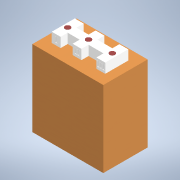
# Autodesk Inventor part: Mesa piezas
Saved by Autodesk Inventor 2020 (Build 240168000, 168)
## iProperties
Created: 2019-10-05
Part Number: Mesa piezas
Material: Genérico
Document SubType Name: Modeling
Designer: dasa1
Density: 1 g/cm^3
Appearance: Valor por defecto
Author: dasa1
Autodesk Inventor part; units mm, degrees
ref_plane "YZ Plane" through (0, 0, 0) normal (1, 0, 0) x (0, 1, 0)
ref_plane "XZ Plane" through (0, 0, 0) normal (0, 1, 0) x (-1, 0, 0)
ref_plane "XY Plane" through (0, 0, 0) normal (0, 0, 1) x (1, 0, 0)
sketch "Boceto1" plane through (0, 0, 0) normal (0, 1, 0) x (-1, 0, 0)
  line L0 (0, 0) -> (800, 0)
  line L1 (800, 0) -> (800, 500)
  line L2 (800, 500) -> (0, 500)
  line L3 (0, 500) -> (0, 0)
  dimension "d0" = 800
  dimension "d1" = 500
  constraints: 8 end point, 2 parallel, 1 horizontal, 1 perpendicular
  measures "d0" distance of L2.end L1.end
  measures "d1" distance of L1.end L0.end
extrude "Extrusión1" add sketch "Boceto1" along normal blind 860
sketch "Boceto2" plane through (0, 860, 0) normal (0, 1, 0) x (1, 0, 0)
  line L0 (-800, 0) -> (-800, -500) construction
  line L1 (-800, -500) -> (0, -500) construction
  line L2 (0, -500) -> (0, 0) construction
  line L3 (0, 0) -> (-800, 0) construction
  line L4 (0, -500) -> (0, 0) construction
  line L5 (0, -250) -> (-800, -250) construction
  line L6 (-800, 0) -> (-800, -500) construction
  line L7 (-800, -250) -> (-651.5, -250) construction
  line L8 (-651.5, -250) -> (-701.5, -250) construction
  line L9 (-701.5, -250) -> (-701.5, -120) construction
  line L10 (-701.5, -120) -> (-651.5, -120) construction
  line L11 (-651.5, -120) -> (-651.5, -250) construction
  line L12 (-651.5, -250) -> (-148.5, -250) construction
  line L13 (-148.5, -250) -> (-98.5, -250) construction
  line L14 (-98.5, -250) -> (-98.5, -380) construction
  line L15 (-98.5, -380) -> (-148.5, -380) construction
  line L16 (-148.5, -380) -> (-148.5, -250) construction
  line L17 (-98.5, -380) -> (-701.5, -380) construction
  line L18 (-701.5, -380) -> (-701.5, -120) construction
  line L19 (-701.5, -120) -> (-98.5, -120) construction
  line L20 (-98.5, -120) -> (-98.5, -380) construction
  line L21 (-651.5, -250) -> (-416.5, -250) construction
  line L22 (-416.5, -250) -> (-148.5, -250) construction
  line L23 (-701.5, -120) -> (-601.5, -120) construction
  line L24 (-601.5, -120) -> (-601.5, -380) construction
  line L25 (-601.5, -380) -> (-701.5, -380) construction
  line L26 (-701.5, -380) -> (-701.5, -120) construction
  line L27 (-416.5, -250) -> (-466.5, -250) construction
  line L28 (-466.5, -250) -> (-466.5, -120) construction
  line L29 (-466.5, -120) -> (-416.5, -120) construction
  line L30 (-416.5, -120) -> (-416.5, -250) construction
  line L31 (-466.5, -120) -> (-366.5, -120) construction
  line L32 (-366.5, -120) -> (-366.5, -380) construction
  line L33 (-366.5, -380) -> (-466.5, -380) construction
  line L34 (-466.5, -380) -> (-466.5, -120) construction
  line L35 (-98.5, -380) -> (-198.5, -380) construction
  line L36 (-198.5, -380) -> (-198.5, -120) construction
  line L37 (-198.5, -120) -> (-98.5, -120) construction
  line L38 (-98.5, -120) -> (-98.5, -380) construction
  line L39 (-701.5, -250) -> (-701.5, -200) construction
  line L40 (-701.5, -200) -> (-98.5, -200) construction
  line L41 (-98.5, -200) -> (-98.5, -300) construction
  line L42 (-98.5, -300) -> (-701.5, -300) construction
  line L43 (-701.5, -300) -> (-701.5, -200) construction
  line L44 (-701.5, -120) -> (-601.5, -120)
  line L45 (-601.5, -120) -> (-601.5, -200)
  line L46 (-601.5, -200) -> (-466.5, -200)
  line L47 (-466.5, -200) -> (-466.5, -120)
  line L48 (-466.5, -120) -> (-366.5, -120)
  line L49 (-366.5, -120) -> (-366.5, -200)
  line L50 (-366.5, -200) -> (-198.5, -200)
  line L51 (-198.5, -200) -> (-198.5, -120)
  line L52 (-198.5, -120) -> (-98.5, -120)
  line L53 (-98.5, -120) -> (-98.5, -380)
  line L54 (-198.5, -380) -> (-98.5, -380)
  line L55 (-198.5, -380) -> (-198.5, -300)
  line L56 (-198.5, -300) -> (-366.5, -300)
  line L57 (-366.5, -300) -> (-366.5, -380)
  line L58 (-366.5, -380) -> (-466.5, -380)
  line L59 (-466.5, -380) -> (-466.5, -300)
  line L60 (-466.5, -300) -> (-601.5, -300)
  line L61 (-601.5, -300) -> (-601.5, -380)
  line L62 (-601.5, -380) -> (-701.5, -380)
  line L63 (-701.5, -380) -> (-701.5, -120)
  dimension "d8" = 148.5
  dimension "d71" = 50
  dimension "d72" = 130
  dimension "d73" = 503
  dimension "d74" = 148.5
  dimension "d75" = 50
  dimension "d76" = 130
  dimension "d77" = 235
  dimension "d78" = 268
  dimension "d79" = 100
  dimension "d80" = 260
  dimension "d81" = 50
  dimension "d82" = 130
  dimension "d83" = 100
  dimension "d84" = 260
  dimension "d85" = 100
  dimension "d86" = 260
  dimension "d87" = 50
  dimension "d88" = 100
  constraints: 116 end point, 21 point on line, 16 parallel, 14 perpendicular, 8 horizontal, 7 collinear, 2 midpoint
  measures "d8" distance of L5.end L7.end
  measures "d71" distance of L9.end L10.end
  measures "d72" distance of L8.end L9.end
  measures "d73" distance of L7.end L12.end
  measures "d74" distance of L5.start L12.end
  measures "d75" distance of L14.end L15.end
  measures "d76" distance of L13.end L14.end
  measures "d77" distance of L7.end L21.end
  measures "d78" distance of L21.end L12.end
  measures "d79" distance of L24.end L25.end
  measures "d80" distance of L23.end L24.end
  measures "d81" distance of L28.end L29.end
  measures "d82" distance of L27.end L28.end
  measures "d83" distance of L32.end L33.end
  measures "d84" distance of L31.end L32.end
  measures "d85" distance of L36.end L37.end
  measures "d86" distance of L35.end L36.end
  measures "d87" distance of L8.end L39.end
  measures "d88" distance of L40.end L41.end
extrude "Extrusión4" add sketch "Boceto2" along normal blind 110
sketch "Boceto5" plane through (-701.5, 860, 380) normal (0, 0, 1) x (1, 0, 0)
  line L0 (100, 0) -> (0, 0) construction
  line L1 (100, 0) -> (100, 110) construction
  line L2 (0, 110) -> (100, 110) construction
  line L3 (0, 0) -> (0, 110) construction
  line L4 (335, 0) -> (235, 0) construction
  line L5 (335, 0) -> (335, 110) construction
  line L6 (235, 110) -> (335, 110) construction
  line L7 (235, 0) -> (235, 110) construction
  line L8 (603, 0) -> (503, 0) construction
  line L9 (603, 0) -> (603, 110) construction
  line L10 (503, 110) -> (603, 110) construction
  line L11 (503, 0) -> (503, 110) construction
  line L12 (100, 110) -> (0, 110) construction
  line L13 (603, 0) -> (603, 110) construction
  line L14 (0, 110) -> (603, 110) construction
  line L15 (603, 110) -> (603, 85) construction
  line L16 (603, 85) -> (0, 85) construction
  line L17 (0, 85) -> (0, 110) construction
  line L18 (0, 0) -> (0, 110) construction
  line L19 (603, 0) -> (0, 0) construction
  line L20 (0, 0) -> (0, 25) construction
  line L21 (0, 25) -> (603, 25) construction
  line L22 (603, 25) -> (603, 0) construction
  line L23 (50, 25) -> (50, 85) construction
  line L24 (285, 25) -> (285, 85) construction
  line L25 (553, 25) -> (553, 85) construction
  line L26 (50, 25) -> (35, 25) construction
  line L27 (35, 25) -> (35, 26)
  line L28 (39, 30) -> (41, 30)
  line L29 (50, 30) -> (50, 25) construction
  line L30 (50, 25) -> (45, 25) construction
  line L31 (45, 34) -> (45, 76)
  line L32 (45, 85) -> (50, 85) construction
  line L33 (50, 85) -> (50, 25) construction
  line L34 (50, 85) -> (35, 85) construction
  line L35 (35, 85) -> (35, 84)
  line L36 (39, 80) -> (41, 80)
  line L37 (50, 80) -> (50, 85) construction
  arc A0 (45, 76) -> (41, 80) centre (41, 76) ccw
  arc A1 (35, 84) -> (39, 80) centre (39, 84) ccw
  arc A2 (41, 30) -> (45, 34) centre (41, 34) ccw
  arc A3 (39, 30) -> (35, 26) centre (39, 26) ccw
  line L38 (35, 85) -> (50, 85)
  line L39 (35, 25) -> (50, 25)
  line L40 (50, 25) -> (65, 25) construction
  line L41 (65, 25) -> (65, 26)
  line L42 (61, 30) -> (59, 30)
  line L43 (50, 25) -> (55, 25) construction
  line L44 (55, 34) -> (55, 76)
  line L45 (55, 85) -> (50, 85) construction
  line L46 (50, 85) -> (65, 85) construction
  line L47 (65, 85) -> (65, 84)
  line L48 (61, 80) -> (59, 80)
  arc A4 (59, 80) -> (55, 76) centre (59, 76) ccw
  arc A5 (61, 80) -> (65, 84) centre (61, 84) ccw
  arc A6 (55, 34) -> (59, 30) centre (59, 34) ccw
  arc A7 (65, 26) -> (61, 30) centre (61, 26) ccw
  line L49 (65, 85) -> (50, 85)
  line L50 (65, 25) -> (50, 25)
  line L51 (553, 25) -> (553, 85) construction
  line L52 (553, 25) -> (538, 25) construction
  line L53 (538, 25) -> (538, 26)
  line L54 (542, 30) -> (544, 30)
  line L55 (553, 30) -> (553, 25) construction
  line L56 (553, 25) -> (548, 25) construction
  line L57 (548, 34) -> (548, 76)
  line L58 (548, 85) -> (553, 85) construction
  line L59 (553, 85) -> (553, 25) construction
  line L60 (553, 85) -> (538, 85) construction
  line L61 (538, 85) -> (538, 84)
  line L62 (542, 80) -> (544, 80)
  line L63 (553, 80) -> (553, 85) construction
  arc A8 (548, 76) -> (544, 80) centre (544, 76) ccw
  arc A9 (538, 84) -> (542, 80) centre (542, 84) ccw
  arc A10 (544, 30) -> (548, 34) centre (544, 34) ccw
  arc A11 (542, 30) -> (538, 26) centre (542, 26) ccw
  line L64 (538, 85) -> (553, 85)
  line L65 (538, 25) -> (553, 25)
  line L66 (558, 34) -> (558, 76)
  line L67 (553, 25) -> (558, 25) construction
  arc A12 (558, 34) -> (562, 30) centre (562, 34) ccw
  line L68 (564, 30) -> (562, 30)
  line L69 (568, 25) -> (568, 26)
  line L70 (553, 25) -> (568, 25) construction
  line L71 (568, 25) -> (553, 25)
  arc A13 (568, 26) -> (564, 30) centre (564, 26) ccw
  arc A14 (562, 80) -> (558, 76) centre (562, 76) ccw
  line L72 (564, 80) -> (562, 80)
  arc A15 (564, 80) -> (568, 84) centre (564, 84) ccw
  line L73 (558, 85) -> (553, 85) construction
  line L74 (553, 85) -> (568, 85) construction
  line L75 (568, 85) -> (553, 85)
  line L76 (568, 85) -> (568, 84)
  line L77 (300, 25) -> (300, 85) construction
  line L78 (300, 25) -> (285, 25) construction
  line L79 (285, 25) -> (285, 26)
  line L80 (289, 30) -> (291, 30)
  line L81 (300, 30) -> (300, 25) construction
  line L82 (300, 25) -> (295, 25) construction
  line L83 (295, 34) -> (295, 76)
  line L84 (295, 85) -> (300, 85) construction
  line L85 (300, 85) -> (300, 25) construction
  line L86 (300, 85) -> (285, 85) construction
  line L87 (285, 85) -> (285, 84)
  line L88 (289, 80) -> (291, 80)
  line L89 (300, 80) -> (300, 85) construction
  arc A16 (295, 76) -> (291, 80) centre (291, 76) ccw
  arc A17 (285, 84) -> (289, 80) centre (289, 84) ccw
  arc A18 (291, 30) -> (295, 34) centre (291, 34) ccw
  arc A19 (289, 30) -> (285, 26) centre (289, 26) ccw
  line L90 (285, 85) -> (300, 85)
  line L91 (285, 25) -> (300, 25)
  line L92 (305, 34) -> (305, 76)
  line L93 (300, 25) -> (305, 25) construction
  arc A20 (305, 34) -> (309, 30) centre (309, 34) ccw
  line L94 (311, 30) -> (309, 30)
  line L95 (315, 25) -> (315, 26)
  line L96 (300, 25) -> (315, 25) construction
  line L97 (315, 25) -> (300, 25)
  arc A21 (315, 26) -> (311, 30) centre (311, 26) ccw
  arc A22 (309, 80) -> (305, 76) centre (309, 76) ccw
  line L98 (311, 80) -> (309, 80)
  arc A23 (311, 80) -> (315, 84) centre (311, 84) ccw
  line L99 (305, 85) -> (300, 85) construction
  line L100 (300, 85) -> (315, 85) construction
  line L101 (315, 85) -> (300, 85)
  line L102 (315, 85) -> (315, 84)
  line L103 (583, 25) -> (583, 85) construction
  line L104 (583, 25) -> (568, 25) construction
  line L105 (568, 25) -> (568, 26)
  line L106 (572, 30) -> (574, 30)
  line L107 (583, 30) -> (583, 25) construction
  line L108 (583, 25) -> (578, 25) construction
  line L109 (578, 34) -> (578, 76)
  line L110 (578, 85) -> (583, 85) construction
  line L111 (583, 85) -> (583, 25) construction
  line L112 (583, 85) -> (568, 85) construction
  line L113 (568, 85) -> (568, 84)
  line L114 (572, 80) -> (574, 80)
  line L115 (583, 80) -> (583, 85) construction
  arc A24 (578, 76) -> (574, 80) centre (574, 76) ccw
  arc A25 (568, 84) -> (572, 80) centre (572, 84) ccw
  arc A26 (574, 30) -> (578, 34) centre (574, 34) ccw
  arc A27 (572, 30) -> (568, 26) centre (572, 26) ccw
  line L116 (568, 85) -> (583, 85)
  line L117 (568, 25) -> (583, 25)
  line L118 (588, 34) -> (588, 76)
  line L119 (583, 25) -> (588, 25) construction
  arc A28 (588, 34) -> (592, 30) centre (592, 34) ccw
  line L120 (594, 30) -> (592, 30)
  line L121 (598, 25) -> (598, 26)
  line L122 (583, 25) -> (598, 25) construction
  line L123 (598, 25) -> (583, 25)
  arc A29 (598, 26) -> (594, 30) centre (594, 26) ccw
  arc A30 (592, 80) -> (588, 76) centre (592, 76) ccw
  line L124 (594, 80) -> (592, 80)
  arc A31 (594, 80) -> (598, 84) centre (594, 84) ccw
  line L125 (588, 85) -> (583, 85) construction
  line L126 (583, 85) -> (598, 85) construction
  line L127 (598, 85) -> (583, 85)
  line L128 (598, 85) -> (598, 84)
  line L129 (270, 25) -> (270, 85) construction
  line L130 (270, 25) -> (255, 25) construction
  line L131 (255, 25) -> (255, 26)
  line L132 (259, 30) -> (261, 30)
  line L133 (270, 30) -> (270, 25) construction
  line L134 (270, 25) -> (265, 25) construction
  line L135 (265, 34) -> (265, 76)
  line L136 (265, 85) -> (270, 85) construction
  line L137 (270, 85) -> (270, 25) construction
  line L138 (270, 85) -> (255, 85) construction
  line L139 (255, 85) -> (255, 84)
  line L140 (259, 80) -> (261, 80)
  line L141 (270, 80) -> (270, 85) construction
  arc A32 (265, 76) -> (261, 80) centre (261, 76) ccw
  arc A33 (255, 84) -> (259, 80) centre (259, 84) ccw
  arc A34 (261, 30) -> (265, 34) centre (261, 34) ccw
  arc A35 (259, 30) -> (255, 26) centre (259, 26) ccw
  line L142 (255, 85) -> (270, 85)
  line L143 (255, 25) -> (270, 25)
  line L144 (275, 34) -> (275, 76)
  line L145 (270, 25) -> (275, 25) construction
  arc A36 (275, 34) -> (279, 30) centre (279, 34) ccw
  line L146 (281, 30) -> (279, 30)
  line L147 (285, 25) -> (285, 26)
  line L148 (270, 25) -> (285, 25) construction
  line L149 (285, 25) -> (270, 25)
  arc A37 (285, 26) -> (281, 30) centre (281, 26) ccw
  arc A38 (279, 80) -> (275, 76) centre (279, 76) ccw
  line L150 (281, 80) -> (279, 80)
  arc A39 (281, 80) -> (285, 84) centre (281, 84) ccw
  line L151 (275, 85) -> (270, 85) construction
  line L152 (270, 85) -> (285, 85) construction
  line L153 (285, 85) -> (270, 85)
  line L154 (285, 85) -> (285, 84)
  line L155 (523, 25) -> (523, 85) construction
  line L156 (523, 25) -> (508, 25) construction
  line L157 (508, 25) -> (508, 26)
  line L158 (512, 30) -> (514, 30)
  line L159 (523, 30) -> (523, 25) construction
  line L160 (523, 25) -> (518, 25) construction
  line L161 (518, 34) -> (518, 76)
  line L162 (518, 85) -> (523, 85) construction
  line L163 (523, 85) -> (523, 25) construction
  line L164 (523, 85) -> (508, 85) construction
  line L165 (508, 85) -> (508, 84)
  line L166 (512, 80) -> (514, 80)
  line L167 (523, 80) -> (523, 85) construction
  arc A40 (518, 76) -> (514, 80) centre (514, 76) ccw
  arc A41 (508, 84) -> (512, 80) centre (512, 84) ccw
  arc A42 (514, 30) -> (518, 34) centre (514, 34) ccw
  arc A43 (512, 30) -> (508, 26) centre (512, 26) ccw
  line L168 (508, 85) -> (523, 85)
  line L169 (508, 25) -> (523, 25)
  line L170 (528, 34) -> (528, 76)
  line L171 (523, 25) -> (528, 25) construction
  arc A44 (528, 34) -> (532, 30) centre (532, 34) ccw
  line L172 (534, 30) -> (532, 30)
  line L173 (538, 25) -> (538, 26)
  line L174 (523, 25) -> (538, 25) construction
  line L175 (538, 25) -> (523, 25)
  arc A45 (538, 26) -> (534, 30) centre (534, 26) ccw
  arc A46 (532, 80) -> (528, 76) centre (532, 76) ccw
  line L176 (534, 80) -> (532, 80)
  arc A47 (534, 80) -> (538, 84) centre (534, 84) ccw
  line L177 (528, 85) -> (523, 85) construction
  line L178 (523, 85) -> (538, 85) construction
  line L179 (538, 85) -> (523, 85)
  line L180 (538, 85) -> (538, 84)
  point P0 (701.5, -860)
  point P1 (35, 30)
  point P2 (35, 80)
  point P3 (65, 30)
  point P4 (65, 80)
  point P5 (538, 30)
  point P6 (538, 80)
  point P7 (568, 30)
  point P8 (568, 80)
  point P9 (285, 30)
  point P10 (285, 80)
  point P11 (315, 30)
  point P12 (315, 80)
  point P13 (568, 30)
  point P14 (568, 80)
  point P15 (598, 30)
  point P16 (598, 80)
  point P17 (255, 30)
  point P18 (255, 80)
  point P19 (285, 30)
  point P20 (285, 80)
  point P21 (508, 30)
  point P22 (508, 80)
  point P23 (538, 30)
  point P24 (538, 80)
  point P25 (568, 26)
  point P26 (568, 84)
  point P27 (538, 84)
  point P28 (538, 26)
  point P29 (285, 26)
  point P30 (285, 84)
  dimension "d91" = 110
  dimension "d92" = 25
  dimension "d93" = 25
  dimension "d94" = 15
  dimension "d95" = 5
  dimension "d96" = 5
  dimension "d97" = 15
  dimension "d98" = 5
  dimension "d99" = 4
  dimension "d100" = 35
  dimension "d101" = 15
  dimension "d102" = 5
  dimension "d103" = 5
  dimension "d104" = 15
  dimension "d105" = 5
  dimension "d106" = 4
  dimension "d107" = 15
  dimension "d108" = 5
  dimension "d109" = 5
  dimension "d110" = 15
  dimension "d111" = 5
  dimension "d112" = 4
  dimension "d113" = 15
  dimension "d114" = 5
  dimension "d115" = 5
  dimension "d116" = 15
  dimension "d117" = 5
  dimension "d118" = 4
  dimension "d119" = 15
  dimension "d120" = 5
  dimension "d121" = 5
  dimension "d122" = 15
  dimension "d123" = 5
  dimension "d124" = 4
  dimension "d125" = 15
  dimension "d126" = 5
  dimension "d127" = 5
  dimension "d128" = 15
  dimension "d129" = 5
  dimension "d130" = 4
  constraints: 332 end point, 108 symmetric about line, 105 point on line, 96 point on circle, 48 centre point, 48 tangent, 40 parallel, 23 perpendicular, 20 horizontal, 18 equal radius, 12 collinear, 24 other
  measures "d91" distance of L8.start L9.end
  measures "d92" distance of L14.end L15.end
  measures "d93" distance of L19.end L20.end
  measures "d94" distance of point (35, 30) L29.start
  measures "d95" distance of L26.end point (35, 30)
  measures "d96" distance of L32.start L32.end
  measures "d97" distance of L37.start point (35, 80)
  measures "d98" distance of point (35, 80) L34.end
  measures "d99" radius of A0
  measures "d100" distance of L20.end L26.end
  measures "d101" distance of point (538, 30) L55.start
  measures "d102" distance of L52.end point (538, 30)
  measures "d103" distance of L58.start L59.start
  measures "d104" distance of L63.start point (538, 80)
  measures "d105" distance of point (538, 80) L60.end
  measures "d106" radius of A8
  measures "d107" distance of point (285, 30) L81.start
  measures "d108" distance of L78.end point (285, 30)
  measures "d109" distance of L84.start L85.start
  measures "d110" distance of L89.start point (285, 80)
  measures "d111" distance of point (285, 80) L86.end
  measures "d112" radius of A16
  measures "d113" distance of point (568, 30) L107.start
  measures "d114" distance of L104.end point (568, 30)
  measures "d115" distance of L110.start L111.start
  measures "d116" distance of L115.start point (568, 80)
  measures "d117" distance of point (568, 80) L112.end
  measures "d118" radius of A24
  measures "d119" distance of point (255, 30) L133.start
  measures "d120" distance of L130.end point (255, 30)
  measures "d121" distance of L136.start L137.start
  measures "d122" distance of L141.start point (255, 80)
  measures "d123" distance of point (255, 80) L138.end
  measures "d124" radius of A32
  measures "d125" distance of point (508, 30) L159.start
  measures "d126" distance of L156.end point (508, 30)
  measures "d127" distance of L162.start L163.start
  measures "d128" distance of L167.start point (508, 80)
  measures "d129" distance of point (508, 80) L164.end
  measures "d130" radius of A40
extrude "Extrusión5" cut sketch "Boceto5" against normal blind 260 contours L27 A3 L28 A2 L31 A0 L36 A1 L35 L38 L49 L47 A5 L48 A4 L44 A6 L42 A7 L41 L50 L39 | L175 L169 L157 A43 L158 A42 L161 A40 L166 A41 L165 L168 L179 L61 A47 L176 A46 L170 A44 L172 A45 L53 | L53 A11 L54 A10 L57 A8 L62 A9 L61 L64 L75 L76 A15 L72 A14 L66 A12 L68 A13 L69 L71 L65 | L69 A27 L106 A26 L109 A24 L114 A25 L76 L116 L127 L128 A31 L124 A30 L118 A28 L120 A29 L121 L123 L117 | L149 L143 L131 A35 L132 A34 L135 A32 L140 A33 L139 L142 L153 L87 A39 L150 A38 L144 A36 L146 A37 L79 | L79 A19 L80 A18 L83 A16 L88 A17 L87 L90 L101 L102 A23 L98 A22 L92 A20 L94 A21 L95 L97 L91
sketch "Boceto6" plane through (0, 970, 0) normal (0, 1, 0) x (1, 0, 0)
  line L0 (-601.5, -120) -> (-601.5, -200) construction
  line L1 (-601.5, -200) -> (-466.5, -200) construction
  line L2 (-466.5, -200) -> (-466.5, -120) construction
  line L3 (-466.5, -120) -> (-366.5, -120) construction
  line L4 (-366.5, -120) -> (-366.5, -200) construction
  line L5 (-366.5, -200) -> (-198.5, -200) construction
  line L6 (-198.5, -200) -> (-198.5, -120) construction
  line L7 (-198.5, -120) -> (-98.5, -120) construction
  line L8 (-98.5, -120) -> (-98.5, -380) construction
  line L9 (-98.5, -380) -> (-198.5, -380) construction
  line L10 (-198.5, -380) -> (-198.5, -300) construction
  line L11 (-198.5, -300) -> (-366.5, -300) construction
  line L12 (-366.5, -300) -> (-366.5, -380) construction
  line L13 (-366.5, -380) -> (-466.5, -380) construction
  line L14 (-466.5, -380) -> (-466.5, -300) construction
  line L15 (-466.5, -300) -> (-601.5, -300) construction
  line L16 (-601.5, -300) -> (-601.5, -380) construction
  line L17 (-601.5, -380) -> (-701.5, -380) construction
  line L18 (-701.5, -380) -> (-701.5, -120) construction
  line L19 (-701.5, -120) -> (-601.5, -120) construction
  line L20 (0, 0) -> (-800, 0) construction
  line L21 (-800, 0) -> (-800, -500) construction
  line L22 (-800, -500) -> (0, -500) construction
  line L23 (0, -500) -> (0, 0) construction
  line L24 (-701.5, -120) -> (-701.5, -380) construction
  line L25 (-701.5, -250) -> (-651.5, -250) construction
  line L26 (-651.5, -250) -> (-416.5, -250) construction
  line L27 (-646.5, -380) -> (-646.5, -120) construction
  line L28 (-651.5, -250) -> (-416.5, -250) construction
  line L29 (-416.5, -250) -> (-148.5, -250) construction
  circle A0 centre (-148.5, -250) radius 30
  circle A1 centre (-416.5, -250) radius 30
  circle A2 centre (-651.5, -250) radius 30
  dimension "d133" = 50
  dimension "d134" = 235
  dimension "d135" = 0
  dimension "d136" = 268
  dimension "d137" = 60
  dimension "d138" = 60
  dimension "d139" = 60
  constraints: 8 end point, 3 centre point, 3 coincident, 2 horizontal, 1 collinear, 1 midpoint, 1 perpendicular, 1 point on line
  measures "d133" distance of L25.start L25.end
  measures "d134" distance of L25.end L26.end
  measures "d135" distance between parallel lines of L26 L28
  measures "d136" distance of L26.end L29.end
  measures "d137" diameter of A0
  measures "d138" diameter of A1
  measures "d139" diameter of A2
extrude "Extrusión6" add sketch "Boceto6" along normal blind 3
